Autodesk Fusion 360 part; units mm, degrees
(part 10 of 14)
  line L6515 (-678.1717, -219.075) -> (-667.1732, -219.075)
  line L6516 (-661.6739, -209.55) -> (-667.1732, -200.025)
  line L6517 (-667.1732, -219.075) -> (-661.6739, -209.55)
  line L6518 (-647.9258, -188.9125) -> (-658.9243, -188.9125)
  line L6519 (-658.9243, -188.9125) -> (-664.4235, -198.4375)
  line L6520 (-664.4235, -198.4375) -> (-658.9243, -207.9625)
  line L6521 (-658.9243, -207.9625) -> (-647.9258, -207.9625)
  line L6522 (-642.4265, -198.4375) -> (-647.9258, -188.9125)
  line L6523 (-647.9258, -207.9625) -> (-642.4265, -198.4375)
  line L6524 (-628.6783, -177.8) -> (-639.6769, -177.8)
  line L6525 (-639.6769, -177.8) -> (-645.1761, -187.325)
  line L6526 (-645.1761, -187.325) -> (-639.6769, -196.85)
  line L6527 (-639.6769, -196.85) -> (-628.6783, -196.85)
  line L6528 (-623.1791, -187.325) -> (-628.6783, -177.8)
  line L6529 (-628.6783, -196.85) -> (-623.1791, -187.325)
  line L6530 (-609.4309, -166.6875) -> (-620.4295, -166.6875)
  line L6531 (-620.4295, -166.6875) -> (-625.9287, -176.2125)
  line L6532 (-625.9287, -176.2125) -> (-620.4295, -185.7375)
  line L6533 (-620.4295, -185.7375) -> (-609.4309, -185.7375)
  line L6534 (-603.9317, -176.2125) -> (-609.4309, -166.6875)
  line L6535 (-609.4309, -185.7375) -> (-603.9317, -176.2125)
  line L6536 (-590.1835, -155.575) -> (-601.182, -155.575)
  line L6537 (-601.182, -155.575) -> (-606.6813, -165.1)
  line L6538 (-606.6813, -165.1) -> (-601.182, -174.625)
  line L6539 (-601.182, -174.625) -> (-590.1835, -174.625)
  line L6540 (-584.6843, -165.1) -> (-590.1835, -155.575)
  line L6541 (-590.1835, -174.625) -> (-584.6843, -165.1)
  line L6542 (-570.9361, -144.4625) -> (-581.9346, -144.4625)
  line L6543 (-581.9346, -144.4625) -> (-587.4339, -153.9875)
  line L6544 (-587.4339, -153.9875) -> (-581.9346, -163.5125)
  line L6545 (-581.9346, -163.5125) -> (-570.9361, -163.5125)
  line L6546 (-565.4368, -153.9875) -> (-570.9361, -144.4625)
  line L6547 (-570.9361, -163.5125) -> (-565.4368, -153.9875)
  line L6548 (-551.6887, -133.35) -> (-562.6872, -133.35)
  line L6549 (-562.6872, -133.35) -> (-568.1865, -142.875)
  line L6550 (-568.1865, -142.875) -> (-562.6872, -152.4)
  line L6551 (-562.6872, -152.4) -> (-551.6887, -152.4)
  line L6552 (-546.1894, -142.875) -> (-551.6887, -133.35)
  line L6553 (-551.6887, -152.4) -> (-546.1894, -142.875)
  line L6554 (-532.4413, -122.2375) -> (-543.4398, -122.2375)
  line L6555 (-543.4398, -122.2375) -> (-548.9391, -131.7625)
  line L6556 (-548.9391, -131.7625) -> (-543.4398, -141.2875)
  line L6557 (-543.4398, -141.2875) -> (-532.4413, -141.2875)
  line L6558 (-526.942, -131.7625) -> (-532.4413, -122.2375)
  line L6559 (-532.4413, -141.2875) -> (-526.942, -131.7625)
  line L6560 (-513.1939, -111.125) -> (-524.1924, -111.125)
  line L6561 (-524.1924, -111.125) -> (-529.6916, -120.65)
  line L6562 (-529.6916, -120.65) -> (-524.1924, -130.175)
  line L6563 (-524.1924, -130.175) -> (-513.1939, -130.175)
  line L6564 (-507.6946, -120.65) -> (-513.1939, -111.125)
  line L6565 (-513.1939, -130.175) -> (-507.6946, -120.65)
  line L6566 (-493.9464, -100.0125) -> (-504.945, -100.0125)
  line L6567 (-504.945, -100.0125) -> (-510.4442, -109.5375)
  line L6568 (-510.4442, -109.5375) -> (-504.945, -119.0625)
  line L6569 (-504.945, -119.0625) -> (-493.9464, -119.0625)
  line L6570 (-488.4472, -109.5375) -> (-493.9464, -100.0125)
  line L6571 (-493.9464, -119.0625) -> (-488.4472, -109.5375)
  line L6572 (-474.699, -88.9) -> (-485.6976, -88.9)
  line L6573 (-485.6976, -88.9) -> (-491.1968, -98.425)
  line L6574 (-491.1968, -98.425) -> (-485.6976, -107.95)
  line L6575 (-485.6976, -107.95) -> (-474.699, -107.95)
  line L6576 (-469.1998, -98.425) -> (-474.699, -88.9)
  line L6577 (-474.699, -107.95) -> (-469.1998, -98.425)
  line L6578 (-455.4516, -77.7875) -> (-466.4501, -77.7875)
  line L6579 (-466.4501, -77.7875) -> (-471.9494, -87.3125)
  line L6580 (-471.9494, -87.3125) -> (-466.4501, -96.8375)
  line L6581 (-466.4501, -96.8375) -> (-455.4516, -96.8375)
  line L6582 (-449.9524, -87.3125) -> (-455.4516, -77.7875)
  line L6583 (-455.4516, -96.8375) -> (-449.9524, -87.3125)
  line L6584 (-436.2042, -66.675) -> (-447.2027, -66.675)
  line L6585 (-447.2027, -66.675) -> (-452.702, -76.2)
  line L6586 (-452.702, -76.2) -> (-447.2027, -85.725)
  line L6587 (-447.2027, -85.725) -> (-436.2042, -85.725)
  line L6588 (-430.7049, -76.2) -> (-436.2042, -66.675)
  line L6589 (-436.2042, -85.725) -> (-430.7049, -76.2)
  line L6590 (-416.9568, -55.5625) -> (-427.9553, -55.5625)
  line L6591 (-427.9553, -55.5625) -> (-433.4546, -65.0875)
  line L6592 (-433.4546, -65.0875) -> (-427.9553, -74.6125)
  line L6593 (-427.9553, -74.6125) -> (-416.9568, -74.6125)
  line L6594 (-411.4575, -65.0875) -> (-416.9568, -55.5625)
  line L6595 (-416.9568, -74.6125) -> (-411.4575, -65.0875)
  line L6596 (-397.7094, -44.45) -> (-408.7079, -44.45)
  line L6597 (-408.7079, -44.45) -> (-414.2072, -53.975)
  line L6598 (-414.2072, -53.975) -> (-408.7079, -63.5)
  line L6599 (-408.7079, -63.5) -> (-397.7094, -63.5)
  line L6600 (-392.2101, -53.975) -> (-397.7094, -44.45)
  line L6601 (-397.7094, -63.5) -> (-392.2101, -53.975)
  line L6602 (-378.462, -33.3375) -> (-389.4605, -33.3375)
  line L6603 (-389.4605, -33.3375) -> (-394.9597, -42.8625)
  line L6604 (-394.9597, -42.8625) -> (-389.4605, -52.3875)
  line L6605 (-389.4605, -52.3875) -> (-378.462, -52.3875)
  line L6606 (-372.9627, -42.8625) -> (-378.462, -33.3375)
  line L6607 (-378.462, -52.3875) -> (-372.9627, -42.8625)
  line L6608 (-359.2145, -22.225) -> (-370.2131, -22.225)
  line L6609 (-370.2131, -22.225) -> (-375.7123, -31.75)
  line L6610 (-375.7123, -31.75) -> (-370.2131, -41.275)
  line L6611 (-370.2131, -41.275) -> (-359.2145, -41.275)
  line L6612 (-353.7153, -31.75) -> (-359.2145, -22.225)
  line L6613 (-359.2145, -41.275) -> (-353.7153, -31.75)
  line L6614 (-339.9671, -11.1125) -> (-350.9657, -11.1125)
  line L6615 (-350.9657, -11.1125) -> (-356.4649, -20.6375)
  line L6616 (-356.4649, -20.6375) -> (-350.9657, -30.1625)
  line L6617 (-350.9657, -30.1625) -> (-339.9671, -30.1625)
  line L6618 (-334.4679, -20.6375) -> (-339.9671, -11.1125)
  line L6619 (-339.9671, -30.1625) -> (-334.4679, -20.6375)
  line L6620 (-320.7197, 0) -> (-331.7182, 0)
  line L6621 (-331.7182, 0) -> (-337.2175, -9.525)
  line L6622 (-337.2175, -9.525) -> (-331.7182, -19.05)
  line L6623 (-331.7182, -19.05) -> (-320.7197, -19.05)
  line L6624 (-315.2205, -9.525) -> (-320.7197, 0)
  line L6625 (-320.7197, -19.05) -> (-315.2205, -9.525)
  line L6626 (-301.4723, 11.1125) -> (-312.4708, 11.1125)
  line L6627 (-312.4708, 11.1125) -> (-317.9701, 1.5875)
  line L6628 (-317.9701, 1.5875) -> (-312.4708, -7.9375)
  line L6629 (-312.4708, -7.9375) -> (-301.4723, -7.9375)
  line L6630 (-295.973, 1.5875) -> (-301.4723, 11.1125)
  line L6631 (-301.4723, -7.9375) -> (-295.973, 1.5875)
  line L6632 (-282.2249, 22.225) -> (-293.2234, 22.225)
  line L6633 (-293.2234, 22.225) -> (-298.7227, 12.7)
  line L6634 (-298.7227, 12.7) -> (-293.2234, 3.175)
  line L6635 (-293.2234, 3.175) -> (-282.2249, 3.175)
  line L6636 (-276.7256, 12.7) -> (-282.2249, 22.225)
  line L6637 (-282.2249, 3.175) -> (-276.7256, 12.7)
  line L6638 (-262.9775, 33.3375) -> (-273.976, 33.3375)
  line L6639 (-273.976, 33.3375) -> (-279.4753, 23.8125)
  line L6640 (-279.4753, 23.8125) -> (-273.976, 14.2875)
  line L6641 (-273.976, 14.2875) -> (-262.9775, 14.2875)
  line L6642 (-257.4782, 23.8125) -> (-262.9775, 33.3375)
  line L6643 (-262.9775, 14.2875) -> (-257.4782, 23.8125)
  line L6644 (-243.7301, 44.45) -> (-254.7286, 44.45)
  line L6645 (-254.7286, 44.45) -> (-260.2278, 34.925)
  line L6646 (-260.2278, 34.925) -> (-254.7286, 25.4)
  line L6647 (-254.7286, 25.4) -> (-243.7301, 25.4)
  line L6648 (-238.2308, 34.925) -> (-243.7301, 44.45)
  line L6649 (-243.7301, 25.4) -> (-238.2308, 34.925)
  line L6650 (-224.4826, 55.5625) -> (-235.4812, 55.5625)
  line L6651 (-235.4812, 55.5625) -> (-240.9804, 46.0375)
  line L6652 (-240.9804, 46.0375) -> (-235.4812, 36.5125)
  line L6653 (-235.4812, 36.5125) -> (-224.4826, 36.5125)
  line L6654 (-218.9834, 46.0375) -> (-224.4826, 55.5625)
  line L6655 (-224.4826, 36.5125) -> (-218.9834, 46.0375)
  line L6656 (-205.2352, 66.675) -> (-216.2337, 66.675)
  line L6657 (-216.2337, 66.675) -> (-221.733, 57.15)
  line L6658 (-221.733, 57.15) -> (-216.2337, 47.625)
  line L6659 (-216.2337, 47.625) -> (-205.2352, 47.625)
  line L6660 (-199.736, 57.15) -> (-205.2352, 66.675)
  line L6661 (-205.2352, 47.625) -> (-199.736, 57.15)
  line L6662 (-185.9878, 77.7875) -> (-196.9863, 77.7875)
  line L6663 (-196.9863, 77.7875) -> (-202.4856, 68.2625)
  line L6664 (-202.4856, 68.2625) -> (-196.9863, 58.7375)
  line L6665 (-196.9863, 58.7375) -> (-185.9878, 58.7375)
  line L6666 (-180.4886, 68.2625) -> (-185.9878, 77.7875)
  line L6667 (-185.9878, 58.7375) -> (-180.4886, 68.2625)
  line L6668 (-166.7404, 88.9) -> (-177.7389, 88.9)
  line L6669 (-177.7389, 88.9) -> (-183.2382, 79.375)
  line L6670 (-183.2382, 79.375) -> (-177.7389, 69.85)
  line L6671 (-177.7389, 69.85) -> (-166.7404, 69.85)
  line L6672 (-161.2411, 79.375) -> (-166.7404, 88.9)
  line L6673 (-166.7404, 69.85) -> (-161.2411, 79.375)
  line L6674 (-147.493, 100.0125) -> (-158.4915, 100.0125)
  line L6675 (-158.4915, 100.0125) -> (-163.9908, 90.4875)
  line L6676 (-163.9908, 90.4875) -> (-158.4915, 80.9625)
  line L6677 (-158.4915, 80.9625) -> (-147.493, 80.9625)
  line L6678 (-141.9937, 90.4875) -> (-147.493, 100.0125)
  line L6679 (-147.493, 80.9625) -> (-141.9937, 90.4875)
  line L6680 (-128.2456, 111.125) -> (-139.2441, 111.125)
  line L6681 (-139.2441, 111.125) -> (-144.7434, 101.6)
  line L6682 (-144.7434, 101.6) -> (-139.2441, 92.075)
  line L6683 (-139.2441, 92.075) -> (-128.2456, 92.075)
  line L6684 (-122.7463, 101.6) -> (-128.2456, 111.125)
  line L6685 (-128.2456, 92.075) -> (-122.7463, 101.6)
  line L6686 (-108.9982, 122.2375) -> (-119.9967, 122.2375)
  line L6687 (-119.9967, 122.2375) -> (-125.4959, 112.7125)
  line L6688 (-125.4959, 112.7125) -> (-119.9967, 103.1875)
  line L6689 (-119.9967, 103.1875) -> (-108.9982, 103.1875)
  line L6690 (-103.4989, 112.7125) -> (-108.9982, 122.2375)
  line L6691 (-108.9982, 103.1875) -> (-103.4989, 112.7125)
  line L6692 (-89.7507, 133.35) -> (-100.7493, 133.35)
  line L6693 (-100.7493, 133.35) -> (-106.2485, 123.825)
  line L6694 (-106.2485, 123.825) -> (-100.7493, 114.3)
  line L6695 (-100.7493, 114.3) -> (-89.7507, 114.3)
  line L6696 (-84.2515, 123.825) -> (-89.7507, 133.35)
  line L6697 (-89.7507, 114.3) -> (-84.2515, 123.825)
  line L6698 (-70.5033, 144.4625) -> (-81.5018, 144.4625)
  line L6699 (-81.5018, 144.4625) -> (-87.0011, 134.9375)
  line L6700 (-87.0011, 134.9375) -> (-81.5018, 125.4125)
  line L6701 (-81.5018, 125.4125) -> (-70.5033, 125.4125)
  line L6702 (-65.0041, 134.9375) -> (-70.5033, 144.4625)
  line L6703 (-70.5033, 125.4125) -> (-65.0041, 134.9375)
  line L6704 (-51.2559, 155.575) -> (-62.2544, 155.575)
  line L6705 (-62.2544, 155.575) -> (-67.7537, 146.05)
  line L6706 (-67.7537, 146.05) -> (-62.2544, 136.525)
  line L6707 (-62.2544, 136.525) -> (-51.2559, 136.525)
  line L6708 (-45.7566, 146.05) -> (-51.2559, 155.575)
  line L6709 (-51.2559, 136.525) -> (-45.7566, 146.05)
  line L6710 (-32.0085, 166.6875) -> (-43.007, 166.6875)
  line L6711 (-43.007, 166.6875) -> (-48.5063, 157.1625)
  line L6712 (-48.5063, 157.1625) -> (-43.007, 147.6375)
  line L6713 (-43.007, 147.6375) -> (-32.0085, 147.6375)
  line L6714 (-26.5092, 157.1625) -> (-32.0085, 166.6875)
  line L6715 (-32.0085, 147.6375) -> (-26.5092, 157.1625)
  line L6716 (-12.7611, 177.8) -> (-23.7596, 177.8)
  line L6717 (-23.7596, 177.8) -> (-29.2589, 168.275)
  line L6718 (-29.2589, 168.275) -> (-23.7596, 158.75)
  line L6719 (-23.7596, 158.75) -> (-12.7611, 158.75)
  line L6720 (-7.2618, 168.275) -> (-12.7611, 177.8)
  line L6721 (-12.7611, 158.75) -> (-7.2618, 168.275)
  line L6722 (6.4863, 188.9125) -> (-4.5122, 188.9125)
  line L6723 (-4.5122, 188.9125) -> (-10.0114, 179.3875)
  line L6724 (-10.0114, 179.3875) -> (-4.5122, 169.8625)
  line L6725 (-4.5122, 169.8625) -> (6.4863, 169.8625)
  line L6726 (11.9856, 179.3875) -> (6.4863, 188.9125)
  line L6727 (6.4863, 169.8625) -> (11.9856, 179.3875)
  line L6728 (25.7337, 200.025) -> (14.7352, 200.025)
  line L6729 (14.7352, 200.025) -> (9.236, 190.5)
  line L6730 (9.236, 190.5) -> (14.7352, 180.975)
  line L6731 (14.7352, 180.975) -> (25.7337, 180.975)
  line L6732 (31.233, 190.5) -> (25.7337, 200.025)
  line L6733 (25.7337, 180.975) -> (31.233, 190.5)
  line L6734 (44.9812, 211.1375) -> (33.9826, 211.1375)
  line L6735 (33.9826, 211.1375) -> (28.4834, 201.6125)
  line L6736 (28.4834, 201.6125) -> (33.9826, 192.0875)
  line L6737 (33.9826, 192.0875) -> (44.9812, 192.0875)
  line L6738 (50.4804, 201.6125) -> (44.9812, 211.1375)
  line L6739 (44.9812, 192.0875) -> (50.4804, 201.6125)
  line L6740 (64.2286, 222.25) -> (53.2301, 222.25)
  line L6741 (53.2301, 222.25) -> (47.7308, 212.725)
  line L6742 (47.7308, 212.725) -> (53.2301, 203.2)
  line L6743 (53.2301, 203.2) -> (64.2286, 203.2)
  line L6744 (69.7278, 212.725) -> (64.2286, 222.25)
  line L6745 (64.2286, 203.2) -> (69.7278, 212.725)
  line L6746 (83.476, 233.3625) -> (72.4775, 233.3625)
  line L6747 (72.4775, 233.3625) -> (66.9782, 223.8375)
  line L6748 (66.9782, 223.8375) -> (72.4775, 214.3125)
  line L6749 (72.4775, 214.3125) -> (83.476, 214.3125)
  line L6750 (88.9753, 223.8375) -> (83.476, 233.3625)
  line L6751 (83.476, 214.3125) -> (88.9753, 223.8375)
  line L6752 (102.7234, 244.475) -> (91.7249, 244.475)
  line L6753 (91.7249, 244.475) -> (86.2256, 234.95)
  line L6754 (86.2256, 234.95) -> (91.7249, 225.425)
  line L6755 (91.7249, 225.425) -> (102.7234, 225.425)
  line L6756 (108.2227, 234.95) -> (102.7234, 244.475)
  line L6757 (102.7234, 225.425) -> (108.2227, 234.95)
  line L6758 (121.9708, 255.5875) -> (110.9723, 255.5875)
  line L6759 (110.9723, 255.5875) -> (105.473, 246.0625)
  line L6760 (105.473, 246.0625) -> (110.9723, 236.5375)
  line L6761 (110.9723, 236.5375) -> (121.9708, 236.5375)
  line L6762 (127.4701, 246.0625) -> (121.9708, 255.5875)
  line L6763 (121.9708, 236.5375) -> (127.4701, 246.0625)
  line L6764 (141.2182, 266.7) -> (130.2197, 266.7)
  line L6765 (130.2197, 266.7) -> (124.7205, 257.175)
  line L6766 (124.7205, 257.175) -> (130.2197, 247.65)
  line L6767 (130.2197, 247.65) -> (141.2182, 247.65)
  line L6768 (146.7175, 257.175) -> (141.2182, 266.7)
  line L6769 (141.2182, 247.65) -> (146.7175, 257.175)
  line L6770 (160.4657, 277.8125) -> (149.4671, 277.8125)
  line L6771 (149.4671, 277.8125) -> (143.9679, 268.2875)
  line L6772 (143.9679, 268.2875) -> (149.4671, 258.7625)
  line L6773 (149.4671, 258.7625) -> (160.4657, 258.7625)
  line L6774 (165.9649, 268.2875) -> (160.4657, 277.8125)
  line L6775 (160.4657, 258.7625) -> (165.9649, 268.2875)
  line L6776 (179.7131, 288.925) -> (168.7145, 288.925)
  line L6777 (168.7145, 288.925) -> (163.2153, 279.4)
  line L6778 (163.2153, 279.4) -> (168.7145, 269.875)
  line L6779 (168.7145, 269.875) -> (179.7131, 269.875)
  line L6780 (185.2123, 279.4) -> (179.7131, 288.925)
  line L6781 (179.7131, 269.875) -> (185.2123, 279.4)
  line L6782 (198.9605, 300.0375) -> (187.962, 300.0375)
  line L6783 (187.962, 300.0375) -> (182.4627, 290.5125)
  line L6784 (182.4627, 290.5125) -> (187.962, 280.9875)
  line L6785 (187.962, 280.9875) -> (198.9605, 280.9875)
  line L6786 (204.4597, 290.5125) -> (198.9605, 300.0375)
  line L6787 (198.9605, 280.9875) -> (204.4597, 290.5125)
  line L6788 (218.2079, 311.15) -> (207.2094, 311.15)
  line L6789 (207.2094, 311.15) -> (201.7101, 301.625)
  line L6790 (201.7101, 301.625) -> (207.2094, 292.1)
  line L6791 (207.2094, 292.1) -> (218.2079, 292.1)
  line L6792 (223.7072, 301.625) -> (218.2079, 311.15)
  line L6793 (218.2079, 292.1) -> (223.7072, 301.625)
  line L6794 (237.4553, 322.2625) -> (226.4568, 322.2625)
  line L6795 (226.4568, 322.2625) -> (220.9575, 312.7375)
  line L6796 (220.9575, 312.7375) -> (226.4568, 303.2125)
  line L6797 (226.4568, 303.2125) -> (237.4553, 303.2125)
  line L6798 (242.9546, 312.7375) -> (237.4553, 322.2625)
  line L6799 (237.4553, 303.2125) -> (242.9546, 312.7375)
  line L6800 (256.7027, 333.375) -> (245.7042, 333.375)
  line L6801 (245.7042, 333.375) -> (240.2049, 323.85)
  line L6802 (240.2049, 323.85) -> (245.7042, 314.325)
  line L6803 (245.7042, 314.325) -> (256.7027, 314.325)
  line L6804 (262.202, 323.85) -> (256.7027, 333.375)
  line L6805 (256.7027, 314.325) -> (262.202, 323.85)
  line L6806 (275.9501, 344.4875) -> (264.9516, 344.4875)
  line L6807 (264.9516, 344.4875) -> (259.4524, 334.9625)
  line L6808 (259.4524, 334.9625) -> (264.9516, 325.4375)
  line L6809 (264.9516, 325.4375) -> (275.9501, 325.4375)
  line L6810 (281.4494, 334.9625) -> (275.9501, 344.4875)
  line L6811 (275.9501, 325.4375) -> (281.4494, 334.9625)
  line L6812 (295.1976, 355.6) -> (284.199, 355.6)
  line L6813 (284.199, 355.6) -> (278.6998, 346.075)
  line L6814 (278.6998, 346.075) -> (284.199, 336.55)
  line L6815 (284.199, 336.55) -> (295.1976, 336.55)
  line L6816 (300.6968, 346.075) -> (295.1976, 355.6)
  line L6817 (295.1976, 336.55) -> (300.6968, 346.075)
  line L6818 (314.445, 366.7125) -> (303.4464, 366.7125)
  line L6819 (303.4464, 366.7125) -> (297.9472, 357.1875)
  line L6820 (297.9472, 357.1875) -> (303.4464, 347.6625)
  line L6821 (303.4464, 347.6625) -> (314.445, 347.6625)
  line L6822 (319.9442, 357.1875) -> (314.445, 366.7125)
  line L6823 (314.445, 347.6625) -> (319.9442, 357.1875)
  line L6824 (333.6924, 377.825) -> (322.6939, 377.825)
  line L6825 (322.6939, 377.825) -> (317.1946, 368.3)
  line L6826 (317.1946, 368.3) -> (322.6939, 358.775)
  line L6827 (322.6939, 358.775) -> (333.6924, 358.775)
  line L6828 (339.1916, 368.3) -> (333.6924, 377.825)
  line L6829 (333.6924, 358.775) -> (339.1916, 368.3)
  line L6830 (352.9398, 388.9375) -> (341.9413, 388.9375)
  line L6831 (341.9413, 388.9375) -> (336.442, 379.4125)
  line L6832 (336.442, 379.4125) -> (341.9413, 369.8875)
  line L6833 (341.9413, 369.8875) -> (352.9398, 369.8875)
  line L6834 (358.4391, 379.4125) -> (352.9398, 388.9375)
  line L6835 (352.9398, 369.8875) -> (358.4391, 379.4125)
  line L6836 (372.1872, 400.05) -> (361.1887, 400.05)
  line L6837 (361.1887, 400.05) -> (355.6894, 390.525)
  line L6838 (355.6894, 390.525) -> (361.1887, 381)
  line L6839 (361.1887, 381) -> (372.1872, 381)
  line L6840 (377.6865, 390.525) -> (372.1872, 400.05)
  line L6841 (372.1872, 381) -> (377.6865, 390.525)
  line L6842 (391.4346, 411.1625) -> (380.4361, 411.1625)
  line L6843 (380.4361, 411.1625) -> (374.9368, 401.6375)
  line L6844 (374.9368, 401.6375) -> (380.4361, 392.1125)
  line L6845 (380.4361, 392.1125) -> (391.4346, 392.1125)
  line L6846 (396.9339, 401.6375) -> (391.4346, 411.1625)
  line L6847 (391.4346, 392.1125) -> (396.9339, 401.6375)
  line L6848 (410.682, 422.275) -> (399.6835, 422.275)
  line L6849 (399.6835, 422.275) -> (394.1843, 412.75)
  line L6850 (394.1843, 412.75) -> (399.6835, 403.225)
  line L6851 (399.6835, 403.225) -> (410.682, 403.225)
  line L6852 (416.1813, 412.75) -> (410.682, 422.275)
  line L6853 (410.682, 403.225) -> (416.1813, 412.75)
  line L6854 (-744.1628, -222.25) -> (-755.1614, -222.25)
  line L6855 (-755.1614, -222.25) -> (-760.6606, -231.775)
  line L6856 (-760.6606, -231.775) -> (-755.1614, -241.3)
  line L6857 (-755.1614, -241.3) -> (-744.1628, -241.3)
  line L6858 (-738.6636, -231.775) -> (-744.1628, -222.25)
  line L6859 (-744.1628, -241.3) -> (-738.6636, -231.775)
  line L6860 (-724.9154, -211.1375) -> (-735.9139, -211.1375)
  line L6861 (-735.9139, -211.1375) -> (-741.4132, -220.6625)
  line L6862 (-741.4132, -220.6625) -> (-735.9139, -230.1875)
  line L6863 (-735.9139, -230.1875) -> (-724.9154, -230.1875)
  line L6864 (-719.4162, -220.6625) -> (-724.9154, -211.1375)
  line L6865 (-724.9154, -230.1875) -> (-719.4162, -220.6625)
  line L6866 (-705.668, -200.025) -> (-716.6665, -200.025)
  line L6867 (-716.6665, -200.025) -> (-722.1658, -209.55)
  line L6868 (-722.1658, -209.55) -> (-716.6665, -219.075)
  line L6869 (-716.6665, -219.075) -> (-705.668, -219.075)
  line L6870 (-700.1687, -209.55) -> (-705.668, -200.025)
  line L6871 (-705.668, -219.075) -> (-700.1687, -209.55)
  line L6872 (-686.4206, -188.9125) -> (-697.4191, -188.9125)
  line L6873 (-697.4191, -188.9125) -> (-702.9184, -198.4375)
  line L6874 (-702.9184, -198.4375) -> (-697.4191, -207.9625)
  line L6875 (-697.4191, -207.9625) -> (-686.4206, -207.9625)
  line L6876 (-680.9213, -198.4375) -> (-686.4206, -188.9125)
  line L6877 (-686.4206, -207.9625) -> (-680.9213, -198.4375)
  line L6878 (-667.1732, -177.8) -> (-678.1717, -177.8)
  line L6879 (-678.1717, -177.8) -> (-683.671, -187.325)
  line L6880 (-683.671, -187.325) -> (-678.1717, -196.85)
  line L6881 (-678.1717, -196.85) -> (-667.1732, -196.85)
  line L6882 (-661.6739, -187.325) -> (-667.1732, -177.8)
  line L6883 (-667.1732, -196.85) -> (-661.6739, -187.325)
  line L6884 (-647.9258, -166.6875) -> (-658.9243, -166.6875)
  line L6885 (-658.9243, -166.6875) -> (-664.4235, -176.2125)
  line L6886 (-664.4235, -176.2125) -> (-658.9243, -185.7375)
  line L6887 (-658.9243, -185.7375) -> (-647.9258, -185.7375)
  line L6888 (-642.4265, -176.2125) -> (-647.9258, -166.6875)
  line L6889 (-647.9258, -185.7375) -> (-642.4265, -176.2125)
  line L6890 (-628.6783, -155.575) -> (-639.6769, -155.575)
  line L6891 (-639.6769, -155.575) -> (-645.1761, -165.1)
  line L6892 (-645.1761, -165.1) -> (-639.6769, -174.625)
  line L6893 (-639.6769, -174.625) -> (-628.6783, -174.625)
  line L6894 (-623.1791, -165.1) -> (-628.6783, -155.575)
  line L6895 (-628.6783, -174.625) -> (-623.1791, -165.1)
  line L6896 (-609.4309, -144.4625) -> (-620.4295, -144.4625)
  line L6897 (-620.4295, -144.4625) -> (-625.9287, -153.9875)
  line L6898 (-625.9287, -153.9875) -> (-620.4295, -163.5125)
  line L6899 (-620.4295, -163.5125) -> (-609.4309, -163.5125)
  line L6900 (-603.9317, -153.9875) -> (-609.4309, -144.4625)
  line L6901 (-609.4309, -163.5125) -> (-603.9317, -153.9875)
  line L6902 (-590.1835, -133.35) -> (-601.182, -133.35)
  line L6903 (-601.182, -133.35) -> (-606.6813, -142.875)
  line L6904 (-606.6813, -142.875) -> (-601.182, -152.4)
  line L6905 (-601.182, -152.4) -> (-590.1835, -152.4)
  line L6906 (-584.6843, -142.875) -> (-590.1835, -133.35)
  line L6907 (-590.1835, -152.4) -> (-584.6843, -142.875)
  line L6908 (-570.9361, -122.2375) -> (-581.9346, -122.2375)
  line L6909 (-581.9346, -122.2375) -> (-587.4339, -131.7625)
  line L6910 (-587.4339, -131.7625) -> (-581.9346, -141.2875)
  line L6911 (-581.9346, -141.2875) -> (-570.9361, -141.2875)
  line L6912 (-565.4368, -131.7625) -> (-570.9361, -122.2375)
  line L6913 (-570.9361, -141.2875) -> (-565.4368, -131.7625)
  line L6914 (-551.6887, -111.125) -> (-562.6872, -111.125)
  line L6915 (-562.6872, -111.125) -> (-568.1865, -120.65)
  line L6916 (-568.1865, -120.65) -> (-562.6872, -130.175)
  line L6917 (-562.6872, -130.175) -> (-551.6887, -130.175)
  line L6918 (-546.1894, -120.65) -> (-551.6887, -111.125)
  line L6919 (-551.6887, -130.175) -> (-546.1894, -120.65)
  line L6920 (-532.4413, -100.0125) -> (-543.4398, -100.0125)
  line L6921 (-543.4398, -100.0125) -> (-548.9391, -109.5375)
  line L6922 (-548.9391, -109.5375) -> (-543.4398, -119.0625)
  line L6923 (-543.4398, -119.0625) -> (-532.4413, -119.0625)
  line L6924 (-526.942, -109.5375) -> (-532.4413, -100.0125)
  line L6925 (-532.4413, -119.0625) -> (-526.942, -109.5375)
  line L6926 (-513.1939, -88.9) -> (-524.1924, -88.9)
  line L6927 (-524.1924, -88.9) -> (-529.6916, -98.425)
  line L6928 (-529.6916, -98.425) -> (-524.1924, -107.95)
  line L6929 (-524.1924, -107.95) -> (-513.1939, -107.95)
  line L6930 (-507.6946, -98.425) -> (-513.1939, -88.9)
  line L6931 (-513.1939, -107.95) -> (-507.6946, -98.425)
  line L6932 (-493.9464, -77.7875) -> (-504.945, -77.7875)
  line L6933 (-504.945, -77.7875) -> (-510.4442, -87.3125)
  line L6934 (-510.4442, -87.3125) -> (-504.945, -96.8375)
  line L6935 (-504.945, -96.8375) -> (-493.9464, -96.8375)
  line L6936 (-488.4472, -87.3125) -> (-493.9464, -77.7875)
  line L6937 (-493.9464, -96.8375) -> (-488.4472, -87.3125)
  line L6938 (-474.699, -66.675) -> (-485.6976, -66.675)
  line L6939 (-485.6976, -66.675) -> (-491.1968, -76.2)
  line L6940 (-491.1968, -76.2) -> (-485.6976, -85.725)
  line L6941 (-485.6976, -85.725) -> (-474.699, -85.725)
  line L6942 (-469.1998, -76.2) -> (-474.699, -66.675)
  line L6943 (-474.699, -85.725) -> (-469.1998, -76.2)
  line L6944 (-455.4516, -55.5625) -> (-466.4501, -55.5625)
  line L6945 (-466.4501, -55.5625) -> (-471.9494, -65.0875)
  line L6946 (-471.9494, -65.0875) -> (-466.4501, -74.6125)
  line L6947 (-466.4501, -74.6125) -> (-455.4516, -74.6125)
  line L6948 (-449.9524, -65.0875) -> (-455.4516, -55.5625)
  line L6949 (-455.4516, -74.6125) -> (-449.9524, -65.0875)
  line L6950 (-436.2042, -44.45) -> (-447.2027, -44.45)
  line L6951 (-447.2027, -44.45) -> (-452.702, -53.975)
  line L6952 (-452.702, -53.975) -> (-447.2027, -63.5)
  line L6953 (-447.2027, -63.5) -> (-436.2042, -63.5)
  line L6954 (-430.7049, -53.975) -> (-436.2042, -44.45)
  line L6955 (-436.2042, -63.5) -> (-430.7049, -53.975)
  line L6956 (-416.9568, -33.3375) -> (-427.9553, -33.3375)
  line L6957 (-427.9553, -33.3375) -> (-433.4546, -42.8625)
  line L6958 (-433.4546, -42.8625) -> (-427.9553, -52.3875)
  line L6959 (-427.9553, -52.3875) -> (-416.9568, -52.3875)
  line L6960 (-411.4575, -42.8625) -> (-416.9568, -33.3375)
  line L6961 (-416.9568, -52.3875) -> (-411.4575, -42.8625)
  line L6962 (-397.7094, -22.225) -> (-408.7079, -22.225)
  line L6963 (-408.7079, -22.225) -> (-414.2072, -31.75)
  line L6964 (-414.2072, -31.75) -> (-408.7079, -41.275)
  line L6965 (-408.7079, -41.275) -> (-397.7094, -41.275)
  line L6966 (-392.2101, -31.75) -> (-397.7094, -22.225)
  line L6967 (-397.7094, -41.275) -> (-392.2101, -31.75)
  line L6968 (-378.462, -11.1125) -> (-389.4605, -11.1125)
  line L6969 (-389.4605, -11.1125) -> (-394.9597, -20.6375)
  line L6970 (-394.9597, -20.6375) -> (-389.4605, -30.1625)
  line L6971 (-389.4605, -30.1625) -> (-378.462, -30.1625)
  line L6972 (-372.9627, -20.6375) -> (-378.462, -11.1125)
  line L6973 (-378.462, -30.1625) -> (-372.9627, -20.6375)
  line L6974 (-359.2145, 0) -> (-370.2131, 0)
  line L6975 (-370.2131, 0) -> (-375.7123, -9.525)
  line L6976 (-375.7123, -9.525) -> (-370.2131, -19.05)
  line L6977 (-370.2131, -19.05) -> (-359.2145, -19.05)
  line L6978 (-353.7153, -9.525) -> (-359.2145, 0)
  line L6979 (-359.2145, -19.05) -> (-353.7153, -9.525)
  line L6980 (-339.9671, 11.1125) -> (-350.9657, 11.1125)
  line L6981 (-350.9657, 11.1125) -> (-356.4649, 1.5875)
  line L6982 (-356.4649, 1.5875) -> (-350.9657, -7.9375)
  line L6983 (-350.9657, -7.9375) -> (-339.9671, -7.9375)
  line L6984 (-334.4679, 1.5875) -> (-339.9671, 11.1125)
  line L6985 (-339.9671, -7.9375) -> (-334.4679, 1.5875)
  line L6986 (-320.7197, 22.225) -> (-331.7182, 22.225)
  line L6987 (-331.7182, 22.225) -> (-337.2175, 12.7)
  line L6988 (-337.2175, 12.7) -> (-331.7182, 3.175)
  line L6989 (-331.7182, 3.175) -> (-320.7197, 3.175)
  line L6990 (-315.2205, 12.7) -> (-320.7197, 22.225)
  line L6991 (-320.7197, 3.175) -> (-315.2205, 12.7)
  line L6992 (-301.4723, 33.3375) -> (-312.4708, 33.3375)
  line L6993 (-312.4708, 33.3375) -> (-317.9701, 23.8125)
  line L6994 (-317.9701, 23.8125) -> (-312.4708, 14.2875)
  line L6995 (-312.4708, 14.2875) -> (-301.4723, 14.2875)
  line L6996 (-295.973, 23.8125) -> (-301.4723, 33.3375)
  line L6997 (-301.4723, 14.2875) -> (-295.973, 23.8125)
  line L6998 (-282.2249, 44.45) -> (-293.2234, 44.45)
  line L6999 (-293.2234, 44.45) -> (-298.7227, 34.925)
  line L7000 (-298.7227, 34.925) -> (-293.2234, 25.4)
  line L7001 (-293.2234, 25.4) -> (-282.2249, 25.4)
  line L7002 (-276.7256, 34.925) -> (-282.2249, 44.45)
  line L7003 (-282.2249, 25.4) -> (-276.7256, 34.925)
  line L7004 (-262.9775, 55.5625) -> (-273.976, 55.5625)
  line L7005 (-273.976, 55.5625) -> (-279.4753, 46.0375)
  line L7006 (-279.4753, 46.0375) -> (-273.976, 36.5125)
  line L7007 (-273.976, 36.5125) -> (-262.9775, 36.5125)
  line L7008 (-257.4782, 46.0375) -> (-262.9775, 55.5625)
  line L7009 (-262.9775, 36.5125) -> (-257.4782, 46.0375)
  line L7010 (-243.7301, 66.675) -> (-254.7286, 66.675)
  line L7011 (-254.7286, 66.675) -> (-260.2278, 57.15)
  line L7012 (-260.2278, 57.15) -> (-254.7286, 47.625)
  line L7013 (-254.7286, 47.625) -> (-243.7301, 47.625)
  line L7014 (-238.2308, 57.15) -> (-243.7301, 66.675)
  line L7015 (-243.7301, 47.625) -> (-238.2308, 57.15)
  line L7016 (-224.4826, 77.7875) -> (-235.4812, 77.7875)
  line L7017 (-235.4812, 77.7875) -> (-240.9804, 68.2625)
  line L7018 (-240.9804, 68.2625) -> (-235.4812, 58.7375)
  line L7019 (-235.4812, 58.7375) -> (-224.4826, 58.7375)
  line L7020 (-218.9834, 68.2625) -> (-224.4826, 77.7875)
  line L7021 (-224.4826, 58.7375) -> (-218.9834, 68.2625)
  line L7022 (-205.2352, 88.9) -> (-216.2337, 88.9)
  line L7023 (-216.2337, 88.9) -> (-221.733, 79.375)
  line L7024 (-221.733, 79.375) -> (-216.2337, 69.85)
  line L7025 (-216.2337, 69.85) -> (-205.2352, 69.85)
  line L7026 (-199.736, 79.375) -> (-205.2352, 88.9)
  line L7027 (-205.2352, 69.85) -> (-199.736, 79.375)
  line L7028 (-185.9878, 100.0125) -> (-196.9863, 100.0125)
  line L7029 (-196.9863, 100.0125) -> (-202.4856, 90.4875)
  line L7030 (-202.4856, 90.4875) -> (-196.9863, 80.9625)
  line L7031 (-196.9863, 80.9625) -> (-185.9878, 80.9625)
  line L7032 (-180.4886, 90.4875) -> (-185.9878, 100.0125)
  line L7033 (-185.9878, 80.9625) -> (-180.4886, 90.4875)
  line L7034 (-166.7404, 111.125) -> (-177.7389, 111.125)
  line L7035 (-177.7389, 111.125) -> (-183.2382, 101.6)
  line L7036 (-183.2382, 101.6) -> (-177.7389, 92.075)
  line L7037 (-177.7389, 92.075) -> (-166.7404, 92.075)
  line L7038 (-161.2411, 101.6) -> (-166.7404, 111.125)
  line L7039 (-166.7404, 92.075) -> (-161.2411, 101.6)
  line L7040 (-147.493, 122.2375) -> (-158.4915, 122.2375)
  line L7041 (-158.4915, 122.2375) -> (-163.9908, 112.7125)
  line L7042 (-163.9908, 112.7125) -> (-158.4915, 103.1875)
  line L7043 (-158.4915, 103.1875) -> (-147.493, 103.1875)
  line L7044 (-141.9937, 112.7125) -> (-147.493, 122.2375)
  line L7045 (-147.493, 103.1875) -> (-141.9937, 112.7125)
  line L7046 (-128.2456, 133.35) -> (-139.2441, 133.35)
  line L7047 (-139.2441, 133.35) -> (-144.7434, 123.825)
  line L7048 (-144.7434, 123.825) -> (-139.2441, 114.3)
  line L7049 (-139.2441, 114.3) -> (-128.2456, 114.3)
  line L7050 (-122.7463, 123.825) -> (-128.2456, 133.35)
  line L7051 (-128.2456, 114.3) -> (-122.7463, 123.825)
  line L7052 (-108.9982, 144.4625) -> (-119.9967, 144.4625)
  line L7053 (-119.9967, 144.4625) -> (-125.4959, 134.9375)
  line L7054 (-125.4959, 134.9375) -> (-119.9967, 125.4125)
  line L7055 (-119.9967, 125.4125) -> (-108.9982, 125.4125)
  line L7056 (-103.4989, 134.9375) -> (-108.9982, 144.4625)
  line L7057 (-108.9982, 125.4125) -> (-103.4989, 134.9375)
  line L7058 (-89.7507, 155.575) -> (-100.7493, 155.575)
  line L7059 (-100.7493, 155.575) -> (-106.2485, 146.05)
  line L7060 (-106.2485, 146.05) -> (-100.7493, 136.525)
  line L7061 (-100.7493, 136.525) -> (-89.7507, 136.525)
  line L7062 (-84.2515, 146.05) -> (-89.7507, 155.575)
  line L7063 (-89.7507, 136.525) -> (-84.2515, 146.05)
  line L7064 (-70.5033, 166.6875) -> (-81.5018, 166.6875)
  line L7065 (-81.5018, 166.6875) -> (-87.0011, 157.1625)
  line L7066 (-87.0011, 157.1625) -> (-81.5018, 147.6375)
  line L7067 (-81.5018, 147.6375) -> (-70.5033, 147.6375)
  line L7068 (-65.0041, 157.1625) -> (-70.5033, 166.6875)
  line L7069 (-70.5033, 147.6375) -> (-65.0041, 157.1625)
  line L7070 (-51.2559, 177.8) -> (-62.2544, 177.8)
  line L7071 (-62.2544, 177.8) -> (-67.7537, 168.275)
  line L7072 (-67.7537, 168.275) -> (-62.2544, 158.75)
  line L7073 (-62.2544, 158.75) -> (-51.2559, 158.75)
  line L7074 (-45.7566, 168.275) -> (-51.2559, 177.8)
  line L7075 (-51.2559, 158.75) -> (-45.7566, 168.275)
  line L7076 (-32.0085, 188.9125) -> (-43.007, 188.9125)
  line L7077 (-43.007, 188.9125) -> (-48.5063, 179.3875)
  line L7078 (-48.5063, 179.3875) -> (-43.007, 169.8625)
  line L7079 (-43.007, 169.8625) -> (-32.0085, 169.8625)
  line L7080 (-26.5092, 179.3875) -> (-32.0085, 188.9125)
  line L7081 (-32.0085, 169.8625) -> (-26.5092, 179.3875)
  line L7082 (-12.7611, 200.025) -> (-23.7596, 200.025)
  line L7083 (-23.7596, 200.025) -> (-29.2589, 190.5)
  line L7084 (-29.2589, 190.5) -> (-23.7596, 180.975)
  line L7085 (-23.7596, 180.975) -> (-12.7611, 180.975)
  line L7086 (-7.2618, 190.5) -> (-12.7611, 200.025)
  line L7087 (-12.7611, 180.975) -> (-7.2618, 190.5)
  line L7088 (6.4863, 211.1375) -> (-4.5122, 211.1375)
  line L7089 (-4.5122, 211.1375) -> (-10.0114, 201.6125)
  line L7090 (-10.0114, 201.6125) -> (-4.5122, 192.0875)
  line L7091 (-4.5122, 192.0875) -> (6.4863, 192.0875)
  line L7092 (11.9856, 201.6125) -> (6.4863, 211.1375)
  line L7093 (6.4863, 192.0875) -> (11.9856, 201.6125)
  line L7094 (25.7337, 222.25) -> (14.7352, 222.25)
  line L7095 (14.7352, 222.25) -> (9.236, 212.725)
  line L7096 (9.236, 212.725) -> (14.7352, 203.2)
  line L7097 (14.7352, 203.2) -> (25.7337, 203.2)
  line L7098 (31.233, 212.725) -> (25.7337, 222.25)
  line L7099 (25.7337, 203.2) -> (31.233, 212.725)
  line L7100 (44.9812, 233.3625) -> (33.9826, 233.3625)
  line L7101 (33.9826, 233.3625) -> (28.4834, 223.8375)
  line L7102 (28.4834, 223.8375) -> (33.9826, 214.3125)
  line L7103 (33.9826, 214.3125) -> (44.9812, 214.3125)
  line L7104 (50.4804, 223.8375) -> (44.9812, 233.3625)
  line L7105 (44.9812, 214.3125) -> (50.4804, 223.8375)
  line L7106 (64.2286, 244.475) -> (53.2301, 244.475)
  line L7107 (53.2301, 244.475) -> (47.7308, 234.95)
  line L7108 (47.7308, 234.95) -> (53.2301, 225.425)
  line L7109 (53.2301, 225.425) -> (64.2286, 225.425)
  line L7110 (69.7278, 234.95) -> (64.2286, 244.475)
  line L7111 (64.2286, 225.425) -> (69.7278, 234.95)
  line L7112 (83.476, 255.5875) -> (72.4775, 255.5875)
  line L7113 (72.4775, 255.5875) -> (66.9782, 246.0625)
  line L7114 (66.9782, 246.0625) -> (72.4775, 236.5375)
  line L7115 (72.4775, 236.5375) -> (83.476, 236.5375)
  line L7116 (88.9753, 246.0625) -> (83.476, 255.5875)
  line L7117 (83.476, 236.5375) -> (88.9753, 246.0625)
  line L7118 (102.7234, 266.7) -> (91.7249, 266.7)
  line L7119 (91.7249, 266.7) -> (86.2256, 257.175)
  line L7120 (86.2256, 257.175) -> (91.7249, 247.65)
  line L7121 (91.7249, 247.65) -> (102.7234, 247.65)
  line L7122 (108.2227, 257.175) -> (102.7234, 266.7)
  line L7123 (102.7234, 247.65) -> (108.2227, 257.175)
  line L7124 (121.9708, 277.8125) -> (110.9723, 277.8125)
  line L7125 (110.9723, 277.8125) -> (105.473, 268.2875)
  line L7126 (105.473, 268.2875) -> (110.9723, 258.7625)
  line L7127 (110.9723, 258.7625) -> (121.9708, 258.7625)
  line L7128 (127.4701, 268.2875) -> (121.9708, 277.8125)
  line L7129 (121.9708, 258.7625) -> (127.4701, 268.2875)
  line L7130 (141.2182, 288.925) -> (130.2197, 288.925)
  line L7131 (130.2197, 288.925) -> (124.7205, 279.4)
  line L7132 (124.7205, 279.4) -> (130.2197, 269.875)
  line L7133 (130.2197, 269.875) -> (141.2182, 269.875)
  line L7134 (146.7175, 279.4) -> (141.2182, 288.925)
  line L7135 (141.2182, 269.875) -> (146.7175, 279.4)
  line L7136 (160.4657, 300.0375) -> (149.4671, 300.0375)
  line L7137 (149.4671, 300.0375) -> (143.9679, 290.5125)
  line L7138 (143.9679, 290.5125) -> (149.4671, 280.9875)
  line L7139 (149.4671, 280.9875) -> (160.4657, 280.9875)
  line L7140 (165.9649, 290.5125) -> (160.4657, 300.0375)
  line L7141 (160.4657, 280.9875) -> (165.9649, 290.5125)
  line L7142 (179.7131, 311.15) -> (168.7145, 311.15)
  line L7143 (168.7145, 311.15) -> (163.2153, 301.625)
  line L7144 (163.2153, 301.625) -> (168.7145, 292.1)
  line L7145 (168.7145, 292.1) -> (179.7131, 292.1)
  line L7146 (185.2123, 301.625) -> (179.7131, 311.15)
  line L7147 (179.7131, 292.1) -> (185.2123, 301.625)
  line L7148 (198.9605, 322.2625) -> (187.962, 322.2625)
  line L7149 (187.962, 322.2625) -> (182.4627, 312.7375)
  line L7150 (182.4627, 312.7375) -> (187.962, 303.2125)
  line L7151 (187.962, 303.2125) -> (198.9605, 303.2125)
  line L7152 (204.4597, 312.7375) -> (198.9605, 322.2625)
  line L7153 (198.9605, 303.2125) -> (204.4597, 312.7375)
  line L7154 (218.2079, 333.375) -> (207.2094, 333.375)
  line L7155 (207.2094, 333.375) -> (201.7101, 323.85)
  line L7156 (201.7101, 323.85) -> (207.2094, 314.325)
  line L7157 (207.2094, 314.325) -> (218.2079, 314.325)
  line L7158 (223.7072, 323.85) -> (218.2079, 333.375)
  line L7159 (218.2079, 314.325) -> (223.7072, 323.85)
  line L7160 (237.4553, 344.4875) -> (226.4568, 344.4875)
  line L7161 (226.4568, 344.4875) -> (220.9575, 334.9625)
  line L7162 (220.9575, 334.9625) -> (226.4568, 325.4375)
  line L7163 (226.4568, 325.4375) -> (237.4553, 325.4375)
  line L7164 (242.9546, 334.9625) -> (237.4553, 344.4875)
  line L7165 (237.4553, 325.4375) -> (242.9546, 334.9625)
  line L7166 (256.7027, 355.6) -> (245.7042, 355.6)
  line L7167 (245.7042, 355.6) -> (240.2049, 346.075)
  line L7168 (240.2049, 346.075) -> (245.7042, 336.55)
  line L7169 (245.7042, 336.55) -> (256.7027, 336.55)
  line L7170 (262.202, 346.075) -> (256.7027, 355.6)
  line L7171 (256.7027, 336.55) -> (262.202, 346.075)
  line L7172 (275.9501, 366.7125) -> (264.9516, 366.7125)
  line L7173 (264.9516, 366.7125) -> (259.4524, 357.1875)
  line L7174 (259.4524, 357.1875) -> (264.9516, 347.6625)
  line L7175 (264.9516, 347.6625) -> (275.9501, 347.6625)
  line L7176 (281.4494, 357.1875) -> (275.9501, 366.7125)
  line L7177 (275.9501, 347.6625) -> (281.4494, 357.1875)
  line L7178 (295.1976, 377.825) -> (284.199, 377.825)
  line L7179 (284.199, 377.825) -> (278.6998, 368.3)
  line L7180 (278.6998, 368.3) -> (284.199, 358.775)
  line L7181 (284.199, 358.775) -> (295.1976, 358.775)
  line L7182 (300.6968, 368.3) -> (295.1976, 377.825)
  line L7183 (295.1976, 358.775) -> (300.6968, 368.3)
  line L7184 (314.445, 388.9375) -> (303.4464, 388.9375)
  line L7185 (303.4464, 388.9375) -> (297.9472, 379.4125)
  line L7186 (297.9472, 379.4125) -> (303.4464, 369.8875)
  line L7187 (303.4464, 369.8875) -> (314.445, 369.8875)
  line L7188 (319.9442, 379.4125) -> (314.445, 388.9375)
  line L7189 (314.445, 369.8875) -> (319.9442, 379.4125)
  line L7190 (333.6924, 400.05) -> (322.6939, 400.05)
  line L7191 (322.6939, 400.05) -> (317.1946, 390.525)
  line L7192 (317.1946, 390.525) -> (322.6939, 381)
  line L7193 (322.6939, 381) -> (333.6924, 381)
  line L7194 (339.1916, 390.525) -> (333.6924, 400.05)
  line L7195 (333.6924, 381) -> (339.1916, 390.525)
  line L7196 (352.9398, 411.1625) -> (341.9413, 411.1625)
  line L7197 (341.9413, 411.1625) -> (336.442, 401.6375)
  line L7198 (336.442, 401.6375) -> (341.9413, 392.1125)
  line L7199 (341.9413, 392.1125) -> (352.9398, 392.1125)
  line L7200 (358.4391, 401.6375) -> (352.9398, 411.1625)
  line L7201 (352.9398, 392.1125) -> (358.4391, 401.6375)
  line L7202 (372.1872, 422.275) -> (361.1887, 422.275)
  line L7203 (361.1887, 422.275) -> (355.6894, 412.75)
  line L7204 (355.6894, 412.75) -> (361.1887, 403.225)
  line L7205 (361.1887, 403.225) -> (372.1872, 403.225)
  line L7206 (377.6865, 412.75) -> (372.1872, 422.275)
  line L7207 (372.1872, 403.225) -> (377.6865, 412.75)
  line L7208 (391.4346, 433.3875) -> (380.4361, 433.3875)
  line L7209 (380.4361, 433.3875) -> (374.9368, 423.8625)
  line L7210 (374.9368, 423.8625) -> (380.4361, 414.3375)
  line L7211 (380.4361, 414.3375) -> (391.4346, 414.3375)
  line L7212 (396.9339, 423.8625) -> (391.4346, 433.3875)
  line L7213 (391.4346, 414.3375) -> (396.9339, 423.8625)
  line L7214 (-763.4102, -211.1375) -> (-774.4088, -211.1375)
  line L7215 (-774.4088, -211.1375) -> (-779.908, -220.6625)
  line L7216 (-779.908, -220.6625) -> (-774.4088, -230.1875)
  line L7217 (-774.4088, -230.1875) -> (-763.4102, -230.1875)
  line L7218 (-757.911, -220.6625) -> (-763.4102, -211.1375)
  line L7219 (-763.4102, -230.1875) -> (-757.911, -220.6625)
  line L7220 (-744.1628, -200.025) -> (-755.1614, -200.025)
  line L7221 (-755.1614, -200.025) -> (-760.6606, -209.55)
  line L7222 (-760.6606, -209.55) -> (-755.1614, -219.075)
  line L7223 (-755.1614, -219.075) -> (-744.1628, -219.075)
  line L7224 (-738.6636, -209.55) -> (-744.1628, -200.025)
  line L7225 (-744.1628, -219.075) -> (-738.6636, -209.55)
  line L7226 (-724.9154, -188.9125) -> (-735.9139, -188.9125)
  line L7227 (-735.9139, -188.9125) -> (-741.4132, -198.4375)
  line L7228 (-741.4132, -198.4375) -> (-735.9139, -207.9625)
  line L7229 (-735.9139, -207.9625) -> (-724.9154, -207.9625)
  line L7230 (-719.4162, -198.4375) -> (-724.9154, -188.9125)
  line L7231 (-724.9154, -207.9625) -> (-719.4162, -198.4375)
  line L7232 (-705.668, -177.8) -> (-716.6665, -177.8)
  line L7233 (-716.6665, -177.8) -> (-722.1658, -187.325)
  line L7234 (-722.1658, -187.325) -> (-716.6665, -196.85)
  line L7235 (-716.6665, -196.85) -> (-705.668, -196.85)
  line L7236 (-700.1687, -187.325) -> (-705.668, -177.8)
  line L7237 (-705.668, -196.85) -> (-700.1687, -187.325)
  line L7238 (-686.4206, -166.6875) -> (-697.4191, -166.6875)
  line L7239 (-697.4191, -166.6875) -> (-702.9184, -176.2125)
  line L7240 (-702.9184, -176.2125) -> (-697.4191, -185.7375)
  line L7241 (-697.4191, -185.7375) -> (-686.4206, -185.7375)
  line L7242 (-680.9213, -176.2125) -> (-686.4206, -166.6875)
  line L7243 (-686.4206, -185.7375) -> (-680.9213, -176.2125)
  line L7244 (-667.1732, -155.575) -> (-678.1717, -155.575)
  line L7245 (-678.1717, -155.575) -> (-683.671, -165.1)
  line L7246 (-683.671, -165.1) -> (-678.1717, -174.625)
  line L7247 (-678.1717, -174.625) -> (-667.1732, -174.625)
  line L7248 (-661.6739, -165.1) -> (-667.1732, -155.575)
  line L7249 (-667.1732, -174.625) -> (-661.6739, -165.1)
  line L7250 (-647.9258, -144.4625) -> (-658.9243, -144.4625)
  line L7251 (-658.9243, -144.4625) -> (-664.4235, -153.9875)
  line L7252 (-664.4235, -153.9875) -> (-658.9243, -163.5125)
  line L7253 (-658.9243, -163.5125) -> (-647.9258, -163.5125)
  line L7254 (-642.4265, -153.9875) -> (-647.9258, -144.4625)
  line L7255 (-647.9258, -163.5125) -> (-642.4265, -153.9875)
  line L7256 (-628.6783, -133.35) -> (-639.6769, -133.35)
  line L7257 (-639.6769, -133.35) -> (-645.1761, -142.875)
  line L7258 (-645.1761, -142.875) -> (-639.6769, -152.4)
  line L7259 (-639.6769, -152.4) -> (-628.6783, -152.4)
  line L7260 (-623.1791, -142.875) -> (-628.6783, -133.35)
  line L7261 (-628.6783, -152.4) -> (-623.1791, -142.875)
  line L7262 (-609.4309, -122.2375) -> (-620.4295, -122.2375)
  line L7263 (-620.4295, -122.2375) -> (-625.9287, -131.7625)
  line L7264 (-625.9287, -131.7625) -> (-620.4295, -141.2875)
  line L7265 (-620.4295, -141.2875) -> (-609.4309, -141.2875)
  line L7266 (-603.9317, -131.7625) -> (-609.4309, -122.2375)
  line L7267 (-609.4309, -141.2875) -> (-603.9317, -131.7625)
  line L7268 (-590.1835, -111.125) -> (-601.182, -111.125)
  line L7269 (-601.182, -111.125) -> (-606.6813, -120.65)
  line L7270 (-606.6813, -120.65) -> (-601.182, -130.175)
  line L7271 (-601.182, -130.175) -> (-590.1835, -130.175)
  line L7272 (-584.6843, -120.65) -> (-590.1835, -111.125)
  line L7273 (-590.1835, -130.175) -> (-584.6843, -120.65)
  line L7274 (-570.9361, -100.0125) -> (-581.9346, -100.0125)
  line L7275 (-581.9346, -100.0125) -> (-587.4339, -109.5375)
  line L7276 (-587.4339, -109.5375) -> (-581.9346, -119.0625)
  line L7277 (-581.9346, -119.0625) -> (-570.9361, -119.0625)
  line L7278 (-565.4368, -109.5375) -> (-570.9361, -100.0125)
  line L7279 (-570.9361, -119.0625) -> (-565.4368, -109.5375)
  line L7280 (-551.6887, -88.9) -> (-562.6872, -88.9)
  line L7281 (-562.6872, -88.9) -> (-568.1865, -98.425)
  line L7282 (-568.1865, -98.425) -> (-562.6872, -107.95)
  line L7283 (-562.6872, -107.95) -> (-551.6887, -107.95)
  line L7284 (-546.1894, -98.425) -> (-551.6887, -88.9)
  line L7285 (-551.6887, -107.95) -> (-546.1894, -98.425)
  line L7286 (-532.4413, -77.7875) -> (-543.4398, -77.7875)
  line L7287 (-543.4398, -77.7875) -> (-548.9391, -87.3125)
  line L7288 (-548.9391, -87.3125) -> (-543.4398, -96.8375)
  line L7289 (-543.4398, -96.8375) -> (-532.4413, -96.8375)
  line L7290 (-526.942, -87.3125) -> (-532.4413, -77.7875)
  line L7291 (-532.4413, -96.8375) -> (-526.942, -87.3125)
  line L7292 (-513.1939, -66.675) -> (-524.1924, -66.675)
  line L7293 (-524.1924, -66.675) -> (-529.6916, -76.2)
  line L7294 (-529.6916, -76.2) -> (-524.1924, -85.725)
  line L7295 (-524.1924, -85.725) -> (-513.1939, -85.725)
  line L7296 (-507.6946, -76.2) -> (-513.1939, -66.675)
  line L7297 (-513.1939, -85.725) -> (-507.6946, -76.2)
  line L7298 (-493.9464, -55.5625) -> (-504.945, -55.5625)
  line L7299 (-504.945, -55.5625) -> (-510.4442, -65.0875)
  line L7300 (-510.4442, -65.0875) -> (-504.945, -74.6125)
  line L7301 (-504.945, -74.6125) -> (-493.9464, -74.6125)
  line L7302 (-488.4472, -65.0875) -> (-493.9464, -55.5625)
  line L7303 (-493.9464, -74.6125) -> (-488.4472, -65.0875)
  line L7304 (-474.699, -44.45) -> (-485.6976, -44.45)
  line L7305 (-485.6976, -44.45) -> (-491.1968, -53.975)
  line L7306 (-491.1968, -53.975) -> (-485.6976, -63.5)
  line L7307 (-485.6976, -63.5) -> (-474.699, -63.5)
  line L7308 (-469.1998, -53.975) -> (-474.699, -44.45)
  line L7309 (-474.699, -63.5) -> (-469.1998, -53.975)
  line L7310 (-455.4516, -33.3375) -> (-466.4501, -33.3375)
  line L7311 (-466.4501, -33.3375) -> (-471.9494, -42.8625)
  line L7312 (-471.9494, -42.8625) -> (-466.4501, -52.3875)
  line L7313 (-466.4501, -52.3875) -> (-455.4516, -52.3875)
  line L7314 (-449.9524, -42.8625) -> (-455.4516, -33.3375)
  line L7315 (-455.4516, -52.3875) -> (-449.9524, -42.8625)
  line L7316 (-436.2042, -22.225) -> (-447.2027, -22.225)
  line L7317 (-447.2027, -22.225) -> (-452.702, -31.75)
  line L7318 (-452.702, -31.75) -> (-447.2027, -41.275)
  line L7319 (-447.2027, -41.275) -> (-436.2042, -41.275)
  line L7320 (-430.7049, -31.75) -> (-436.2042, -22.225)
  line L7321 (-436.2042, -41.275) -> (-430.7049, -31.75)
  line L7322 (-416.9568, -11.1125) -> (-427.9553, -11.1125)
  line L7323 (-427.9553, -11.1125) -> (-433.4546, -20.6375)
  line L7324 (-433.4546, -20.6375) -> (-427.9553, -30.1625)
  line L7325 (-427.9553, -30.1625) -> (-416.9568, -30.1625)
  line L7326 (-411.4575, -20.6375) -> (-416.9568, -11.1125)
  line L7327 (-416.9568, -30.1625) -> (-411.4575, -20.6375)
  line L7328 (-397.7094, 0) -> (-408.7079, 0)
  line L7329 (-408.7079, 0) -> (-414.2072, -9.525)
  line L7330 (-414.2072, -9.525) -> (-408.7079, -19.05)
  line L7331 (-408.7079, -19.05) -> (-397.7094, -19.05)
  line L7332 (-392.2101, -9.525) -> (-397.7094, 0)
  line L7333 (-397.7094, -19.05) -> (-392.2101, -9.525)
  line L7334 (-378.462, 11.1125) -> (-389.4605, 11.1125)
  line L7335 (-389.4605, 11.1125) -> (-394.9597, 1.5875)
  line L7336 (-394.9597, 1.5875) -> (-389.4605, -7.9375)
  line L7337 (-389.4605, -7.9375) -> (-378.462, -7.9375)
  line L7338 (-372.9627, 1.5875) -> (-378.462, 11.1125)
  line L7339 (-378.462, -7.9375) -> (-372.9627, 1.5875)
  line L7340 (-359.2145, 22.225) -> (-370.2131, 22.225)
  line L7341 (-370.2131, 22.225) -> (-375.7123, 12.7)
  line L7342 (-375.7123, 12.7) -> (-370.2131, 3.175)
  line L7343 (-370.2131, 3.175) -> (-359.2145, 3.175)
  line L7344 (-353.7153, 12.7) -> (-359.2145, 22.225)
  line L7345 (-359.2145, 3.175) -> (-353.7153, 12.7)
  line L7346 (-339.9671, 33.3375) -> (-350.9657, 33.3375)
  line L7347 (-350.9657, 33.3375) -> (-356.4649, 23.8125)
  line L7348 (-356.4649, 23.8125) -> (-350.9657, 14.2875)
  line L7349 (-350.9657, 14.2875) -> (-339.9671, 14.2875)
  line L7350 (-334.4679, 23.8125) -> (-339.9671, 33.3375)
  line L7351 (-339.9671, 14.2875) -> (-334.4679, 23.8125)
  line L7352 (-320.7197, 44.45) -> (-331.7182, 44.45)
  line L7353 (-331.7182, 44.45) -> (-337.2175, 34.925)
  line L7354 (-337.2175, 34.925) -> (-331.7182, 25.4)
  line L7355 (-331.7182, 25.4) -> (-320.7197, 25.4)
  line L7356 (-315.2205, 34.925) -> (-320.7197, 44.45)
  line L7357 (-320.7197, 25.4) -> (-315.2205, 34.925)
  line L7358 (-301.4723, 55.5625) -> (-312.4708, 55.5625)
  line L7359 (-312.4708, 55.5625) -> (-317.9701, 46.0375)
  line L7360 (-317.9701, 46.0375) -> (-312.4708, 36.5125)
  line L7361 (-312.4708, 36.5125) -> (-301.4723, 36.5125)
  line L7362 (-295.973, 46.0375) -> (-301.4723, 55.5625)
  line L7363 (-301.4723, 36.5125) -> (-295.973, 46.0375)
  line L7364 (-282.2249, 66.675) -> (-293.2234, 66.675)
  line L7365 (-293.2234, 66.675) -> (-298.7227, 57.15)
  line L7366 (-298.7227, 57.15) -> (-293.2234, 47.625)
  line L7367 (-293.2234, 47.625) -> (-282.2249, 47.625)
  line L7368 (-276.7256, 57.15) -> (-282.2249, 66.675)
  line L7369 (-282.2249, 47.625) -> (-276.7256, 57.15)
  line L7370 (-262.9775, 77.7875) -> (-273.976, 77.7875)
  line L7371 (-273.976, 77.7875) -> (-279.4753, 68.2625)
  line L7372 (-279.4753, 68.2625) -> (-273.976, 58.7375)
  line L7373 (-273.976, 58.7375) -> (-262.9775, 58.7375)
  line L7374 (-257.4782, 68.2625) -> (-262.9775, 77.7875)
  line L7375 (-262.9775, 58.7375) -> (-257.4782, 68.2625)
  line L7376 (-243.7301, 88.9) -> (-254.7286, 88.9)
  line L7377 (-254.7286, 88.9) -> (-260.2278, 79.375)
  line L7378 (-260.2278, 79.375) -> (-254.7286, 69.85)
  line L7379 (-254.7286, 69.85) -> (-243.7301, 69.85)
  line L7380 (-238.2308, 79.375) -> (-243.7301, 88.9)
  line L7381 (-243.7301, 69.85) -> (-238.2308, 79.375)
  line L7382 (-224.4826, 100.0125) -> (-235.4812, 100.0125)
  line L7383 (-235.4812, 100.0125) -> (-240.9804, 90.4875)
  line L7384 (-240.9804, 90.4875) -> (-235.4812, 80.9625)
  line L7385 (-235.4812, 80.9625) -> (-224.4826, 80.9625)
  line L7386 (-218.9834, 90.4875) -> (-224.4826, 100.0125)
  line L7387 (-224.4826, 80.9625) -> (-218.9834, 90.4875)